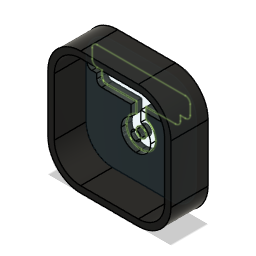
Trellis Keycap blinds open (Autodesk Fusion 360 design; units mm, degrees)
Autodesk Fusion 360 part; units mm, degrees
sketch "Sketch1" plane through (0, 0, 0) normal (0, 0, 1) x (1, 0, 0)
  line L0 (2.72, 5) -> (-2.72, 5)
  line L1 (-5, 2.72) -> (-5, -2.72)
  line L2 (-2.72, -5) -> (2.72, -5)
  line L3 (5, -2.72) -> (5, 2.72)
  line L4 (5, 5) -> (-5, -5) construction
  line L5 (-5, 5) -> (5, -5) construction
  arc A0 (5, 2.72) -> (2.72, 5) centre (2.72, 2.72) ccw
  arc A1 (2.72, -5) -> (5, -2.72) centre (2.72, -2.72) ccw
  arc A2 (-5, -2.72) -> (-2.72, -5) centre (-2.72, -2.72) ccw
  arc A3 (-2.72, 5) -> (-5, 2.72) centre (-2.72, 2.72) ccw
  line L6 (-2.72, -5.2) -> (2.72, -5.2)
  arc A4 (2.72, -5.2) -> (5.2, -2.72) centre (2.72, -2.72) ccw
  line L7 (5.2, -2.72) -> (5.2, 2.72)
  arc A5 (5.2, 2.72) -> (2.72, 5.2) centre (2.72, 2.72) ccw
  line L8 (2.72, 5.2) -> (-2.72, 5.2)
  arc A6 (-2.72, 5.2) -> (-5.2, 2.72) centre (-2.72, 2.72) ccw
  line L9 (-5.2, 2.72) -> (-5.2, -2.72)
  arc A7 (-5.2, -2.72) -> (-2.72, -5.2) centre (-2.72, -2.72) ccw
  line L10 (-2.72, -5.8) -> (2.72, -5.8)
  arc A8 (2.72, -5.8) -> (5.8, -2.72) centre (2.72, -2.72) ccw
  line L11 (5.8, -2.72) -> (5.8, 2.72)
  arc A9 (5.8, 2.72) -> (2.72, 5.8) centre (2.72, 2.72) ccw
  line L12 (2.72, 5.8) -> (-2.72, 5.8)
  arc A10 (-2.72, 5.8) -> (-5.8, 2.72) centre (-2.72, 2.72) ccw
  line L13 (-5.8, 2.72) -> (-5.8, -2.72)
  arc A11 (-5.8, -2.72) -> (-2.72, -5.8) centre (-2.72, -2.72) ccw
  dimension "d1" = 10
  dimension "d2" = 10
  dimension "d3" = 2.28
  dimension "d4" = 0.2
  dimension "d5" = 0.8
  constraint horizontal L0
  constraint perpendicular L0 L1
  constraint parallel L0 L2
  constraint parallel L1 L3
  constraint coincident L4 origin
  constraint coincident L5 origin
  constraint coincident L4.start L0
  constraint coincident L4.start L3
  constraint tangent L0 A0
  constraint tangent L3 A0
  constraint coincident L5.end L3
  constraint coincident L5.end L2
  constraint tangent L3 A1
  constraint tangent L2 A1
  constraint equal A0 A1
  constraint coincident L4.end L2
  constraint coincident L4.end L1
  constraint tangent L2 A2
  constraint tangent L1 A2
  constraint equal A0 A2
  constraint coincident L5.start L1
  constraint coincident L5.start L0
  constraint tangent L1 A3
  constraint tangent L0 A3
  constraint equal A0 A3
  measures "d1" distance of L4.end L5.end
  measures "d2" distance of L5.start L4.end
  measures "d3" radius of A0
extrude "Extrude1" add sketch "Sketch1" along normal blind 3 contours L10 A8 L11 A9 L12 A10 L13 A11 makes body 1
extrude "Extrude2" add sketch "Sketch1" against normal blind 0.5 contours L0 L1 L2 L3 A0 A1 A2 A3 | L6 A4 L7 A5 L8 A6 L9 A7 | L10 A8 L11 A9 L12 A10 L13 A11 bodies 1
sketch "Sketch2" plane through (0, 0, 0) normal (0, 0, 1) x (1, 0, 0)
  line L0 (-2.72, -5.2) -> (2.72, -5.2)
  arc A0 (2.72, -5.2) -> (5.2, -2.72) centre (2.72, -2.72) ccw
  line L1 (5.2, -2.72) -> (5.2, 2.72)
  arc A1 (5.2, 2.72) -> (2.72, 5.2) centre (2.72, 2.72) ccw
  line L2 (2.72, 5.2) -> (-2.72, 5.2)
  arc A2 (-2.72, 5.2) -> (-5.2, 2.72) centre (-2.72, 2.72) ccw
  line L3 (-5.2, 2.72) -> (-5.2, -2.72)
  arc A3 (-5.2, -2.72) -> (-2.72, -5.2) centre (-2.72, -2.72) ccw
  line L4 (-4.1608, 4.0953) -> (4.1574, 4.0953)
  spline S0 degree 3 poles (4.1574, 4.0953) (4.4115, 4.0953) (4.6195, 3.8873) (4.6195, 3.6332) knots 0 0 0 0 1 1 1 1
  line L5 (4.6195, 3.6332) -> (4.6195, 2.7089)
  spline S1 degree 3 poles (4.6195, 2.7089) (4.6195, 2.4548) (4.4115, 2.2468) (4.1574, 2.2468) knots 0 0 0 0 1 1 1 1
  line L6 (4.1574, 2.2468) -> (3.6953, 2.2468)
  line L7 (3.6953, 2.2468) -> (3.6953, 1.7847)
  spline S2 degree 3 poles (3.6953, 1.7847) (3.6953, 1.5305) (3.4873, 1.3226) (3.2331, 1.3226) knots 0 0 0 0 1 1 1 1
  line L8 (3.2331, 1.3226) -> (0.4604, 1.3226)
  line L9 (0.4604, 1.3226) -> (0.4604, 0.3198)
  spline S3 degree 3 poles (0.4604, 0.3198) (1.0011, 0.1303) (1.3847, -0.3873) (1.3847, -0.988) knots 0 0 0 0 1 1 1 1
  spline S4 degree 3 poles (1.3847, -0.988) (1.3847, -1.7552) (0.7654, -2.3744) (-0.0017, -2.3744) knots 0 0 0 0 1 1 1 1
  spline S5 degree 3 poles (-0.0017, -2.3744) (-0.7688, -2.3744) (-1.3881, -1.7552) (-1.3881, -0.988) knots 0 0 0 0 1 1 1 1
  spline S6 degree 3 poles (-1.3881, -0.988) (-1.3881, -0.3827) (-0.9999, 0.1303) (-0.4638, 0.3198) knots 0 0 0 0 1 1 1 1
  line L10 (-0.4638, 0.3198) -> (-0.4638, 1.3226)
  line L11 (-0.4638, 1.3226) -> (-3.2366, 1.3226)
  spline S7 degree 3 poles (-3.2366, 1.3226) (-3.4907, 1.3226) (-3.6987, 1.5305) (-3.6987, 1.7847) knots 0 0 0 0 1 1 1 1
  line L12 (-3.6987, 1.7847) -> (-3.6987, 2.2468)
  line L13 (-3.6987, 2.2468) -> (-4.1608, 2.2468)
  spline S8 degree 3 poles (-4.1608, 2.2468) (-4.415, 2.2468) (-4.6229, 2.4548) (-4.6229, 2.7089) knots 0 0 0 0 1 1 1 1
  line L14 (-4.6229, 2.7089) -> (-4.6229, 3.6332)
  spline S9 degree 3 poles (-4.6229, 3.6332) (-4.6229, 3.8873) (-4.415, 4.0953) (-4.1608, 4.0953) knots 0 0 0 0 1 1 1 1
  spline S10 degree 3 poles (-0.0017, -0.5259) (-0.2559, -0.5259) (-0.4638, -0.7339) (-0.4638, -0.988) knots 0 0 0 0 1 1 1 1
  spline S11 degree 3 poles (-0.4638, -0.988) (-0.4638, -1.2422) (-0.2559, -1.4502) (-0.0017, -1.4502) knots 0 0 0 0 1 1 1 1
  spline S12 degree 3 poles (-0.0017, -1.4502) (0.2525, -1.4502) (0.4604, -1.2422) (0.4604, -0.988) knots 0 0 0 0 1 1 1 1
  spline S13 degree 3 poles (0.4604, -0.988) (0.4604, -0.7339) (0.2525, -0.5259) (-0.0017, -0.5259) knots 0 0 0 0 1 1 1 1
extrude "Extrude3" cut sketch "Sketch2" against normal blind 0.5 contours L4 S0 L5 S1 L6 L7 S2 L8 L9 S3 S4 S5 S6 L10 L11 S7 L12 L13 S8 L14 S9 bodies 1 makes body 2 at (-0.0006, -4.6581, -0.5)
extrude "Extrude4" add sketch "Sketch2" along normal blind 0.5 separate body contours L4 S0 L5 S1 L6 L7 S2 L8 L9 S3 S4 S5 S6 L10 L11 S7 L12 L13 S8 L14 S9 makes body 3
named bodies: "Keycap", "Keycap (1)"
